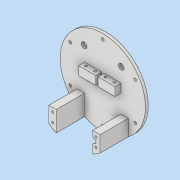
# Autodesk Inventor part: rearServoAttachmentPlate
Saved by Autodesk Inventor 2017 (Build 210142000, 142)
## iProperties
Created: 2016-10-29
Part Number: rearServoAttachmentPlate
Material: ABS Plastic
Document SubType Name: Modeling
Designer: techn
Density: 1.06 g/cm^3
Appearance: Smooth - White
Author: techn
Autodesk Inventor part; units mm, degrees
ref_plane "YZ Plane" through (0, 0, 0) normal (1, 0, 0) x (0, 1, 0)
ref_plane "XZ Plane" through (0, 0, 0) normal (0, 1, 0) x (-1, 0, 0)
ref_plane "XY Plane" through (0, 0, 0) normal (0, 0, 1) x (1, 0, 0)
sketch "Sketch1" plane through (0, 0, 0) normal (0, 0, 1) x (1, 0, 0)
  circle A0 centre (0, 0) radius 47.625
  dimension "d0" = 95.25
  constraints: 1 centre point, 1 coincident
  measures "d0" diameter of A0
extrude "Extrusion1" add sketch "Sketch1" along normal blind 3.175
sketch "Sketch3" plane through (0, 0, 3.175) normal (0, 0, 1) x (1, 0, 0)
  line L0 (1.27, 9.525) -> (20.32, 9.525)
  line L1 (20.32, 9.525) -> (20.32, 0)
  line L2 (20.32, 0) -> (1.27, 0)
  line L3 (1.27, 0) -> (1.27, 9.525)
  line L4 (0, 0) -> (0, -11.0035)
  line L5 (-1.27, 9.525) -> (-20.32, 9.525)
  line L6 (-20.32, 9.525) -> (-20.32, 0)
  line L7 (-20.32, 0) -> (-1.27, 0)
  line L8 (-1.27, 0) -> (-1.27, 9.525)
  dimension "d11" = 19.05
  dimension "d12" = 9.525
  dimension "d13" = 1.27
  dimension "d14" = 0
  constraints: 18 end point, 4 symmetric about line, 2 parallel, 1 horizontal, 1 perpendicular, 1 vertical
  measures "d11" distance of L1.end L2.end
  measures "d12" distance of L0.end L1.end
  measures "d13" distance from line of L3 L4.start
  measures "d14" distance from line of L2 L4.start
extrude "Extrusion3" add sketch "Sketch3" along normal blind 6.604
sketch "Sketch4" plane through (1.27, 9.525, 3.175) normal (0, 1, 0) x (1, 0, 0)
  circle A0 centre (4.445, -2.794) radius 1.27
  line L0 (19.05, -6.604) -> (0, -6.604) projected
  circle A1 centre (14.605, -2.794) radius 1.27
  line L1 (9.525, -6.604) -> (9.525, -7.9119)
  line L2 (-1.27, 3.175) -> (-1.27, 8.3959)
  circle A2 centre (-6.985, -2.794) radius 1.27
  circle A3 centre (-17.145, -2.794) radius 1.27
  dimension "d17" = 2.54
  dimension "d18" = 3.81
  dimension "d19" = 2.54
  dimension "d20" = 3.81
  dimension "d21" = 10.16
  dimension "d22" = 5.08
  constraints: 4 centre point, 4 end point, 2 symmetric about line, 2 vertical, 1 midpoint, 2 other
  measures "d17" diameter of A0
  measures "d18" distance from line of L0 A0.centre
  measures "d19" diameter of A1
  measures "d20" distance from line of L0 A1.centre
  measures "d21" distance of A1.centre A0.centre
  measures "d22" distance from line of L1 A0.centre
extrude "Extrusion4" cut sketch "Sketch4" against normal through all
sketch "Sketch5" plane through (0, 0, 3.175) normal (0, 0, 1) x (1, 0, 0)
  circle A0 centre (20.795, 25.8191) radius 3.175
  line L0 (0, 0) -> (0, 16.9345)
  circle A1 centre (-20.795, 25.8191) radius 3.175
  dimension "d25" = 6.35
  dimension "d26" = 20.795
  dimension "d27" = 25.8191
  constraints: 2 centre point, 2 end point, 1 symmetric about line, 1 vertical, 1 other
  measures "d25" diameter of A0
  measures "d26" horizontal distance of A0.centre L0.start
  measures "d27" vertical distance of A0.centre L0.start
extrude "Extrusion5" cut sketch "Sketch5" against normal blind 25.4
sketch "Sketch6" plane through (0, 0, 3.175) normal (0, 0, 1) x (1, 0, 0)
  line L0 (0, 0) -> (0, 41.91)
  circle A0 centre (0, 41.91) radius 1.5875
  circle A1 centre (-36.2951, 20.955) radius 1.5875
  circle A2 centre (-36.2951, -20.955) radius 1.5875
  circle A3 centre (0, -41.91) radius 1.5875
  circle A4 centre (36.2951, -20.955) radius 1.5875
  circle A5 centre (36.2951, 20.955) radius 1.5875
  dimension "d30" = 41.91
  dimension "d31" = 3.175
  dimension "d34" = 360
  constraints: 6 centre point, 2 end point, 1 coincident, 1 vertical, 13 other
  measures "d30" distance of L0.start L0.end
  measures "d31" diameter of A0
extrude "Extrusion6" cut sketch "Sketch6" against normal blind 25.4
sketch "Sketch7" plane through (0, 0, 3.175) normal (0, 0, 1) x (1, 0, 0)
  line L0 (-28.575, -20.3352) -> (-20.32, -20.3352)
  line L1 (-20.32, -20.3352) -> (-20.32, -43.0725)
  line L2 (-28.575, -38.1) -> (-28.575, -20.3352)
  circle A0 centre (-24.13, -24.6888) radius 1.27
  circle A1 centre (-24.13, -34.8488) radius 1.27
  circle A2 centre (0, 0) radius 47.625 projected
  line L3 (0, 0) -> (0, -12.4863)
  line L4 (28.575, -20.3352) -> (20.32, -20.3352)
  line L5 (20.32, -20.3352) -> (20.32, -43.0725)
  line L6 (28.575, -38.1) -> (28.575, -20.3352)
  circle A3 centre (24.13, -24.6888) radius 1.27
  circle A4 centre (24.13, -34.8488) radius 1.27
  arc A5 (20.32, -43.0725) -> (28.575, -38.1) centre (0, 0) ccw
  dimension "d38" = 20.32
  dimension "d39" = 2.54
  dimension "d40" = 2.54
  dimension "d41" = 24.6888
  dimension "d42" = 10.16
  dimension "d43" = 3.81
  dimension "d44" = 8.255
  constraints: 14 end point, 6 symmetric about line, 5 centre point, 4 point on circle, 1 concentric, 1 horizontal, 1 parallel, 1 perpendicular, 1 vertical, 2 other
  measures "d38" distance from line of point (0, 0) L1
  measures "d39" diameter of A0
  measures "d40" diameter of A1
  measures "d41" vertical distance of A0.centre point (0, 0)
  measures "d42" distance of A0.centre A1.centre
  measures "d43" distance from line of L1 A0.centre
  measures "d44" distance between parallel lines of L1 L2
extrude "Extrusion7" add sketch "Sketch7" along normal blind 31.75 contours L0 L1 A2 L2 | L5 L4 L6 A2
sketch "Sketch8" plane through (0, 0, 34.925) normal (0, 0, 1) x (1, 0, 0)
  circle A0 centre (24.13, -24.6888) radius 1.27 projected
  circle A1 centre (24.13, -34.8488) radius 1.27 projected
  line L0 (20.32, -20.3352) -> (20.32, -43.0725) projected
  line L1 (20.32, -43.0725) -> (20.32, -20.3352) projected
  line L2 (24.13, -31.2293) -> (20.32, -31.2293)
  line L3 (20.32, -31.2293) -> (20.32, -28.0543)
  line L4 (20.32, -28.0543) -> (24.13, -28.0543)
  line L5 (24.13, -28.0543) -> (24.13, -31.2293)
  point P0 (0, 0)
  dimension "d47" = 3.175
  dimension "d48" = 3.3655
  constraints: 8 end point, 2 parallel, 1 horizontal, 1 perpendicular, 1 point on line
  measures "d47" distance between parallel lines of L2 L4
  measures "d48" distance from line of A0.centre L4
extrude "Extrusion8" cut sketch "Sketch8" against normal up to surface (31.75 mm away) contours L4 L5 L2 L0
fillet "Fillet1" radius 3.175 2 edges at (20.32, -28.0543, 19.05) (20.32, -31.2293, 19.05)
body "Solid1"
